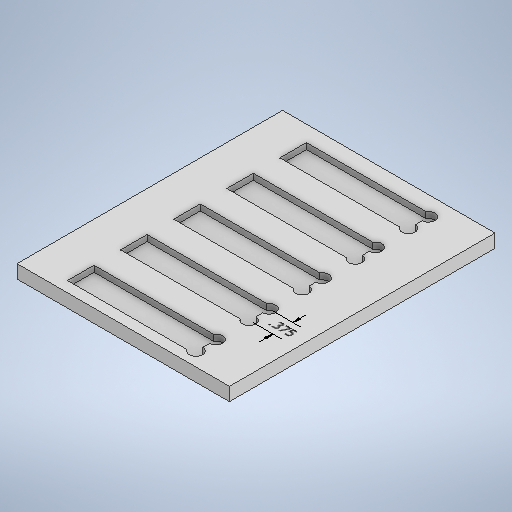
# Autodesk Inventor part: mold plate with alignment
Saved by Autodesk Inventor 2025.3 (Build 293356030, 356C)
## iProperties
Created: 2025-07-30
Part Number: mold plate with alignment
Material: Generic
Document SubType Name: Modeling
Designer: toppe
Density: 1 g/cm^3
Appearance: Default
Author: toppe
Autodesk Inventor part; units mm, degrees
ref_plane "YZ Plane" through (0, 0, 0) normal (1, 0, 0) x (0, 1, 0)
ref_plane "XZ Plane" through (0, 0, 0) normal (0, 1, 0) x (-1, 0, 0)
ref_plane "XY Plane" through (0, 0, 0) normal (0, 0, 1) x (1, 0, 0)
sketch "Sketch1" plane through (0, 0, 0) normal (0, 1, 0) x (-1, 0, 0)
  line L0 (0, 0) -> (101.6, 0)
  line L1 (101.6, 0) -> (101.6, -127)
  line L2 (101.6, -127) -> (0, -127)
  line L3 (0, -127) -> (0, 0)
  dimension "d0" = 101.6
  dimension "d1" = 127
  constraints: 8 end point, 2 parallel, 1 horizontal, 1 perpendicular
  measures "d0" distance of L0.start L0.end
  measures "d1" distance of L2.end L0.start
extrude "Extrusion1" add sketch "Sketch1" along normal blind 6.35
sketch "Sketch2" plane through (0, 6.35, 0) normal (0, 1, 0) x (1, 0, 0)
  line L0 (-82.55, 5.08) -> (-25.4, 5.08)
  line L1 (-22.4915, 9.8367) -> (-22.4915, 13.0117)
  line L2 (-25.3966, 17.78) -> (-82.55, 17.78)
  line L3 (-82.55, 17.78) -> (-82.55, 5.08)
  arc A0 (-25.4, 5.08) -> (-22.4915, 9.8367) centre (-22.6493, 6.6656) ccw
  arc A1 (-22.4915, 13.0117) -> (-25.3966, 17.78) centre (-22.6527, 16.1826) ccw
  line L4 (-101.6, 127) -> (-101.6, 0) projected
  line L5 (-101.6, 0) -> (0, 0) projected
  line L6 (-82.55, 30.48) -> (-25.4, 30.48)
  line L7 (-22.4915, 35.2367) -> (-22.4915, 38.4117)
  line L8 (-25.3966, 43.18) -> (-82.55, 43.18)
  line L9 (-82.55, 43.18) -> (-82.55, 30.48)
  arc A2 (-25.4, 30.48) -> (-22.4915, 35.2367) centre (-22.6493, 32.0656) ccw
  arc A3 (-22.4915, 38.4117) -> (-25.3966, 43.18) centre (-22.6527, 41.5826) ccw
  line L10 (-82.55, 55.88) -> (-25.4, 55.88)
  line L11 (-22.4915, 60.6367) -> (-22.4915, 63.8117)
  line L12 (-25.3966, 68.58) -> (-82.55, 68.58)
  line L13 (-82.55, 68.58) -> (-82.55, 55.88)
  arc A4 (-25.4, 55.88) -> (-22.4915, 60.6367) centre (-22.6493, 57.4656) ccw
  arc A5 (-22.4915, 63.8117) -> (-25.3966, 68.58) centre (-22.6527, 66.9826) ccw
  line L14 (-82.55, 81.28) -> (-25.4, 81.28)
  line L15 (-22.4915, 86.0367) -> (-22.4915, 89.2117)
  line L16 (-25.3966, 93.98) -> (-82.55, 93.98)
  line L17 (-82.55, 93.98) -> (-82.55, 81.28)
  arc A6 (-25.4, 81.28) -> (-22.4915, 86.0367) centre (-22.6493, 82.8656) ccw
  arc A7 (-22.4915, 89.2117) -> (-25.3966, 93.98) centre (-22.6527, 92.3826) ccw
  line L18 (-82.55, 106.68) -> (-25.4, 106.68)
  line L19 (-22.4915, 111.4367) -> (-22.4915, 114.6117)
  line L20 (-25.3966, 119.38) -> (-82.55, 119.38)
  line L21 (-82.55, 119.38) -> (-82.55, 106.68)
  arc A8 (-25.4, 106.68) -> (-22.4915, 111.4367) centre (-22.6493, 108.2656) ccw
  arc A9 (-22.4915, 114.6117) -> (-25.3966, 119.38) centre (-22.6527, 117.7826) ccw
  point P0 (-82.55, 11.43)
  point P1 (-82.55, 36.83)
  point P2 (-82.55, 62.23)
  point P3 (-82.55, 87.63)
  point P4 (-82.55, 113.03)
  dimension "d5" = 12.7
  dimension "d6" = 6.35
  dimension "d7" = 6.35
  dimension "d8" = 3.175
  dimension "d9" = 57.15
  dimension "d10" = 19.05
  dimension "d11" = 5.08
  dimension "d14" = 25.4
  constraints: 40 end point, 20 point on circle, 10 centre point, 2 parallel, 1 horizontal, 1 midpoint, 1 perpendicular, 1 vertical, 60 other
  measures "d5" distance of L2.end L0.start
  measures "d6" diameter of A0
  measures "d7" diameter of A1
  measures "d8" distance of L1.start L1.end
  measures "d9" distance of L0.start L0.end
  measures "d10" distance from line of L4 point (-82.55, 11.43)
  measures "d11" distance between parallel lines of L5 L0
  measures "d14" distance of L0.start L6.start
extrude "Extrusion2" cut sketch "Sketch2" against normal blind 2.921
body "Solid1"
